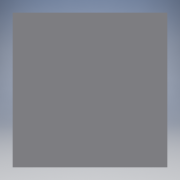
# Autodesk Inventor part: air
Saved by Autodesk Inventor 2018.2 (Build 222227000, 227)
## iProperties
Created: 2018-03-06
Part Number: air
Material: 一般
Document SubType Name: Modeling
Designer: ku_sk
Density: 1 g/cm^3
Appearance: 既定
Author: ku_sk
Autodesk Inventor part; units mm, degrees
ref_plane "YZ Plane" through (0, 0, 0) normal (1, 0, 0) x (0, 1, 0)
ref_plane "XZ Plane" through (0, 0, 0) normal (0, 1, 0) x (-1, 0, 0)
ref_plane "XY Plane" through (0, 0, 0) normal (0, 0, 1) x (1, 0, 0)
sketch "スケッチ1" plane through (0, 0, 0) normal (0, 0, 1) x (1, 0, 0)
  line L0 (-3000, 1000) -> (3000, 1000)
  line L1 (3000, 1000) -> (3000, -1000)
  line L2 (3000, -1000) -> (-3000, -1000)
  line L3 (-3000, -1000) -> (-3000, 1000)
  line L4 (-3000, 1000) -> (3000, -1000) construction
  line L5 (3000, 1000) -> (-3000, -1000) construction
  point P0 (0, 0)
  dimension "d0" = 6000
  dimension "d1" = 2000
  constraints: 12 end point, 2 midpoint, 2 parallel, 1 horizontal, 1 perpendicular
  measures "d0" distance of L0.start L0.end
  measures "d1" distance of L0.end L1.end
extrude "押し出し1" add sketch "スケッチ1" along normal blind 1315 and the other way blind 685
